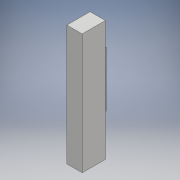
# Autodesk Inventor part: PiezaPuerta-1
Saved by Autodesk Inventor 2017 (Build 210142000, 142)
## iProperties
Created: 2021-02-12
Part Number: PiezaPuerta-1
Material: Generic
Document SubType Name: Modeling
Designer: USUARIO
Density: 1 g/cm^3
Appearance: Default
Author: USUARIO
Autodesk Inventor part; units mm, degrees
ref_plane "YZ Plane" through (0, 0, 0) normal (1, 0, 0) x (0, 1, 0)
ref_plane "XZ Plane" through (0, 0, 0) normal (0, 1, 0) x (-1, 0, 0)
ref_plane "XY Plane" through (0, 0, 0) normal (0, 0, 1) x (1, 0, 0)
sketch "Sketch1" plane through (0, 0, 0) normal (0, 1, 0) x (-1, 0, 0)
  line L0 (0, 0) -> (50.8, 0)
  line L1 (50.8, 0) -> (50.8, -400)
  line L2 (50.8, -400) -> (0, -400)
  line L3 (0, -400) -> (0, 0)
  dimension "d0" = 50.8
  dimension "d1" = 400
  constraints: 8 end point, 2 parallel, 1 horizontal, 1 perpendicular
  measures "d0" distance of L1.end L2.end
  measures "d1" distance of L0.end L1.end
extrude "Extrusion1" add sketch "Sketch1" along normal blind 102.8
sketch "Sketch3" plane through (0, 0, 0) normal (1, 0, 0) x (0, 0, -1)
  line L0 (0, 102.8) -> (101.6, 102.8)
  line L1 (101.6, 102.8) -> (101.6, 77)
  line L2 (101.6, 77) -> (0, 77)
  line L3 (0, 77) -> (0, 102.8)
  line L4 (0, 102.8) -> (400, 102.8) projected
  line L5 (400, 102.8) -> (285, 102.8)
  line L6 (285, 102.8) -> (285, 77)
  line L7 (285, 77) -> (400, 77)
  line L8 (400, 77) -> (400, 102.8)
  point P0 (0, 0)
  dimension "d8" = 101.6
  dimension "d9" = 25.8
  dimension "d10" = 115
  dimension "d11" = 25.8
  constraints: 16 end point, 4 parallel, 2 horizontal, 2 perpendicular
  measures "d8" distance of L1.end L2.end
  measures "d9" distance of L0.end L1.end
  measures "d10" distance of L7.end L6.end
  measures "d11" distance of L6.end L5.end
extrude "Extrusion2" cut sketch "Sketch3" against normal blind 50.8
sketch "Sketch4" plane through (0, 102.8, 0) normal (0, 1, 0) x (1, 0, 0)
  line L0 (0, 101.6) -> (0, 285) projected
  line L1 (0, 285) -> (-50.8, 285) projected
  line L2 (0, 101.6) -> (-23, 101.6)
  line L3 (-23, 101.6) -> (-23, 285)
  line L4 (-23, 285) -> (0, 285)
  line L5 (0, 285) -> (0, 101.6)
  point P0 (0, 0)
  dimension "d14" = 23
  constraints: 8 end point, 2 parallel, 1 horizontal, 1 perpendicular, 1 point on line
  measures "d14" distance of L3.end L4.end
extrude "Extrusion3" cut sketch "Sketch4" against normal blind 25.8
body "Solid1"
